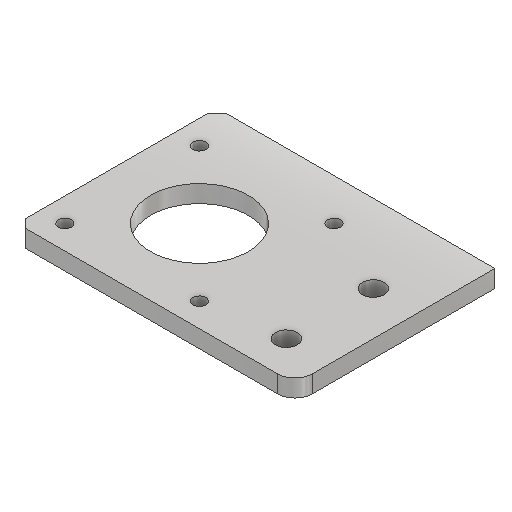
# Autodesk Inventor part: LC_ALU_4mm_Z_Axis_Motor_Mount
Saved by Autodesk Inventor 2026.1 (Build 301233000, 233)
## iProperties
Created: 2017-05-29
Part Number: LC_ALU_4mm_Z_Axis_Motor_Mount
Material: Ogólny
Document SubType Name: Modeling
Designer: Andrzej
Density: 1 g/cm^3
Appearance: Aluminium - polerowane
Mass: 9.89846 g
Surface Area: 63.7259 cm^2
Volume: 9.89846 cm^3
Author: Andrzej
Autodesk Inventor part; units mm, degrees
ref_plane "YZ Plane" through (0, 0, 0) normal (1, 0, 0) x (0, 1, 0)
ref_plane "XZ Plane" through (0, 0, 0) normal (0, 1, 0) x (-1, 0, 0)
ref_plane "XY Plane" through (0, 0, 0) normal (0, 0, 1) x (1, 0, 0)
sketch "Szkic1" plane through (0, 0, 0) normal (0, 0, 1) x (1, 0, 0)
  line L0 (-9.5597, 36.3357) -> (54.4403, 36.3357)
  line L1 (54.4403, 36.3357) -> (54.4403, -9.7143)
  line L2 (54.4403, -9.7143) -> (-9.5597, -9.7143)
  line L3 (-9.5597, -9.7143) -> (-9.5597, 36.3357)
  point P0 (0, 0)
  point P1 (-4.0597, 26.7857)
  point P2 (26.9403, 26.7857)
  point P3 (-4.0597, -4.2143)
  point P4 (26.9403, -4.2143)
  point P5 (11.4403, 11.2857)
  point P6 (44.4403, 18.3357)
  point P7 (44.4403, -1.6893)
  dimension "d0" = 46.05
  dimension "d1" = 64
  dimension "d2" = 15.5
  dimension "d3" = 15.5
  dimension "d4" = 15.5
  dimension "d5" = 15.5
  dimension "d6" = 15.5
  dimension "d7" = 15.5
  dimension "d8" = 15.5
  dimension "d9" = 15.5
  dimension "d11" = 43
  dimension "d12" = 25.05
  dimension "d33" = 10
  dimension "d34" = 10
  dimension "d35" = 8.025
  dimension "d37" = 18
  constraints: 8 end point, 2 parallel, 1 horizontal, 1 perpendicular
  measures "d0" distance of L2.end L0.start
  measures "d1" distance of L1.end L2.end
  measures "d2" horizontal distance of point (11.44, 11.286) point (-4.06, -4.214)
  measures "d3" horizontal distance of point (11.44, 11.286) point (-4.06, -4.214)
  measures "d4" horizontal distance of point (11.44, 11.286) point (-4.06, 26.786)
  measures "d5" horizontal distance of point (11.44, 11.286) point (-4.06, 26.786)
  measures "d6" horizontal distance of point (26.94, 26.786) point (11.44, 11.286)
  measures "d7" horizontal distance of point (11.44, 11.286) point (26.94, 26.786)
  measures "d8" horizontal distance of point (11.44, 11.286) point (26.94, -4.214)
  measures "d9" horizontal distance of point (11.44, 11.286) point (26.94, -4.214)
  measures "d11" distance from line of L1 point (11.44, 11.286)
  measures "d12" distance from line of L0 point (11.44, 11.286)
  measures "d33" distance from line of L1 point (44.44, 18.336)
  measures "d34" distance from line of L1 point (44.44, -1.689)
  measures "d35" distance from line of L2 point (44.44, -1.689)
  measures "d37" distance from line of L0 point (44.44, 18.336)
extrude "Wyciągnięcie proste1" add sketch "Szkic1" along normal blind 4
hole "Otwór1" at (11.4403, 11.2857, 0) direction (0, 0, 1) diameter 22.5 end through all
hole "Otwór2" at (26.9403, -4.2143, 0) at (-4.0597, -4.2143, 0) at (26.9403, 26.7857, 0) at (-4.0597, 26.7857, 0) direction (0, 0, 1) diameter 3 end through all
chamfer "Faza1" distance 2 angle 45 2 edges at (-9.5597, 36.3357, 2) (-9.5597, -9.7143, 2)
fillet "Zaokrąglenie1" radius 4 1 edges at (54.4403, -9.7143, 2)
hole "Otwór3" at (44.4403, 18.3357, 0) at (44.4403, -1.6893, 0) direction (0, 0, 1) diameter 5 end through all
equation "\"d2\" = 0.5 * d10"
equation "\"d3\" = d2"
equation "\"d4\" = d2"
equation "\"d34\" = d33"
equation "\"d10\" = 31"
